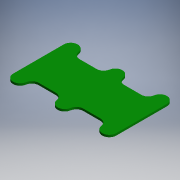
# Autodesk Inventor part: Body_bottom
Saved by Autodesk Inventor 2017 (Build 210142000, 142)
## iProperties
Part Number: Body_bottom
Material: Generic
Document SubType Name: Modeling
Designer: alex-
Appearance: Dark Green
b_mat_thickness: 0,500 cm
b_core_width: 10,000 cm
b_leg_space: 7,500 cm
Author: alex-
Autodesk Inventor part; units mm, degrees
ref_plane "YZ Plane" through (0, 0, 0) normal (1, 0, 0) x (0, 1, 0)
ref_plane "XZ Plane" through (0, 0, 0) normal (0, 1, 0) x (-1, 0, 0)
ref_plane "XY Plane" through (0, 0, 0) normal (0, 0, 1) x (1, 0, 0)
sketch "Sketch1" plane through (0, 0, 0) normal (0, 1, 0) x (-1, 0, 0)
  line L0 (126, 79) -> (92, 79)
  line L1 (126, -79) -> (92, -79)
  line L2 (126, 79) -> (126, -79)
  line L3 (92, 79) -> (92, 50)
  line L4 (92, -50) -> (92, -79)
  line L5 (92, 50) -> (17, 50)
  line L6 (92, -50) -> (17, -50)
  line L7 (17, 50) -> (17, 79)
  line L8 (17, -50) -> (17, -79)
  line L9 (17, 79) -> (-17, 79)
  line L10 (17, -79) -> (-17, -79)
  line L11 (-17, 79) -> (-17, 50)
  line L12 (-17, -50) -> (-17, -79)
  line L13 (-17, 50) -> (-92, 50)
  line L14 (-17, -50) -> (-92, -50)
  line L15 (-92, 50) -> (-92, 79)
  line L16 (-92, -50) -> (-92, -79)
  line L17 (-92, 79) -> (-126, 79)
  line L18 (-92, -79) -> (-126, -79)
  line L19 (-126, 79) -> (-126, -79)
  line L20 (126, 0) -> (-126, 0) construction
  line L21 (0, 79) -> (0, -79) construction
  point P0 (0, 0)
  point P1 (0, 0)
  dimension "d0" = 158
  dimension "b_servo_depth" = 34
  dimension "d3" = 75
  dimension "d4" = 29
  dimension "d5" = 100
  constraints: 44 end point, 16 equal length, 9 vertical, 8 horizontal, 6 horizontal alignment, 5 midpoint, 1 coincident, 1 parallel, 1 perpendicular
  measures "d0" distance of L0.start L1.start
  measures "b_servo_depth" distance of L0.start L0.end
  measures "d3" distance of L3.end L5.end
  measures "d4" distance of L0.end L3.end
  measures "d5" distance between parallel lines of L6 L5
extrude "Extrusion1" add sketch "Sketch1" along normal blind 5
fillet "Fillet1" radius 17 12 edges at (-126, 2.5, 79) (-92, 2.5, 79) (-17, 2.5, 79) (17, 2.5, 79) (92, 2.5, 79) (126, 2.5, 79) (126, 2.5, -79) (92, 2.5, -79) (17, 2.5, -79) (-17, 2.5, -79) (-92, 2.5, -79) (-126, 2.5, -79)
fillet "Fillet2" radius 17 8 edges at (-92, 2.5, 50) (17, 2.5, 50) (-17, 2.5, 50) (92, 2.5, 50) (17, 2.5, -50) (-92, 2.5, -50) (92, 2.5, -50) (-17, 2.5, -50)
equation "\"b_servo_depth\" = sa_diameter + 2 * b_mat_thickness"
equation "\"d3\" = b_leg_space"
equation "\"d4\" = sa_diameter + b_mat_thickness"
equation "\"d5\" = b_core_width"
equation "\"d6\" = b_mat_thickness"
equation "\"d22\" = b_mat_thickness + 0.5 * sa_diameter"
equation "\"d23\" = b_mat_thickness + 0.5 * sa_diameter"
equation "\"b_mat_thickness\" = 5"
equation "\"b_core_width\" = 100"
equation "\"b_leg_space\" = 75"
equation "\"sa_diameter\" = 24"
body "Solid1"
